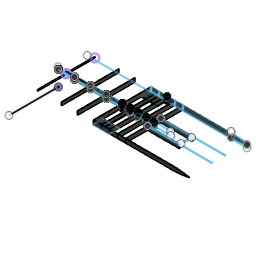
fishtail more cadamaran frame v4 (Autodesk Fusion 360 design; units mm, degrees)
Autodesk Fusion 360 part; units mm, degrees
sketch "Sketch1" plane through (0, 0, 0) normal (0, 1, 0) x (1, 0, 0)
  line L0 (0, 0, 0) -> (0, 0, -1544.9876)
  line L1 (2000, -550) -> (3000, -550)
  spline S0 degree 5 poles (0, -470) (19.8891, -472.7686) (59.6834, -478.151) (119.4225, -485.7607) (199.1707, -494.9751) (299.0134, -504.9326) (399.0022, -513.3461) (499.1108, -520.2801) (599.2925, -525.8722) (699.4727, -530.3612) (799.5726, -534.0348) (899.532, -537.1783) (999.3326, -540.0242) (1099.0214, -542.7014) (1198.7368, -545.1827) (1298.6488, -547.3474) (1398.9006, -549.0438) (1499.5491, -550.1503) (1600.504, -550.6385) (1701.4653, -550.6375) (1802.0225, -550.3661) (1881.8073, -550.1262) (1941.1238, -550.023) (1980.4165, -550) (2000, -550) knots 0 0 0 0 0 0 0.05 0.1 0.15 0.2 0.25 0.3 0.35 0.4 0.45 0.5 0.55 0.6 0.65 0.7 0.75 0.8 0.85 0.9 0.95 1 1 1 1 1 1
  line L2 (1800, -550) -> (2200, -550)
  spline S1 degree 5 poles (2000, -430) (1980.0012, -430) (1940.0021, -429.973) (1879.9994, -429.8512) (1799.9885, -429.5694) (1699.9671, -429.2542) (1599.9436, -429.2586) (1499.9235, -429.829) (1399.91, -431.0929) (1299.9035, -432.9733) (1199.9019, -435.2653) (1099.902, -437.7087) (999.901, -440.0615) (899.8967, -442.1718) (799.8896, -444.0523) (699.8815, -445.8304) (599.8751, -447.701) (499.8734, -449.8794) (399.8791, -452.5548) (299.8937, -455.8432) (199.9182, -459.8058) (119.9458, -463.5341) (59.9712, -466.6451) (19.99, -468.8585) (0, -470) knots 0 0 0 0 0 0 0.05 0.1 0.15 0.2 0.25 0.3 0.35 0.4 0.45 0.5 0.55 0.6 0.65 0.7 0.75 0.8 0.85 0.9 0.95 1 1 1 1 1 1
  line L3 (2204.0501, -430) -> (1795.9499, -430)
  line L4 (2000, -430) -> (3000, -430)
  line L5 (3000, -550) -> (3000, -430)
  point P0 (1500, -430)
  point P1 (500, -450)
  point P2 (500, -520)
  point P3 (1000, -540)
  point P4 (1500, -550)
  point P5 (1000, -440)
  constraint midpoint L1.start L2
  constraint midpoint S1.start L3
  constraint perpendicular L4 L5
  constraint coincident S0.start S1.end
extrude "Extrude1" add sketch "Sketch1" along normal mid plane 20 makes body 1
sketch "Sketch2" plane through (0, -10, 0) normal (0, -1, 0) x (1, 0, 0)
  spline S0 degree 5 poles (0, 470) (19.99, 468.8585) (59.9712, 466.6451) (119.9458, 463.5341) (199.9182, 459.8058) (299.8937, 455.8432) (399.8791, 452.5548) (499.8734, 449.8794) (599.8751, 447.701) (699.8815, 445.8304) (799.8896, 444.0523) (899.8967, 442.1718) (999.901, 440.0615) (1099.902, 437.7087) (1199.9019, 435.2653) (1299.9035, 432.9733) (1399.91, 431.0929) (1499.9235, 429.829) (1599.9436, 429.2586) (1699.9671, 429.2542) (1799.9885, 429.5694) (1879.9994, 429.8512) (1940.0021, 429.973) (1980.0012, 430) (2000, 430) knots -1 -1 -1 -1 -1 -1 -0.95 -0.9 -0.85 -0.8 -0.75 -0.7 -0.65 -0.6 -0.55 -0.5 -0.45 -0.4 -0.35 -0.3 -0.25 -0.2 -0.15 -0.1 -0.05 0 0 0 0 0 0
  line L0 (2000, 430) -> (3000, 430)
  line L1 (3000, 430) -> (3000, 550)
  line L2 (3000, 550) -> (2000, 550)
  spline S1 degree 5 poles (2000, 550) (1980.4165, 550) (1941.1238, 550.023) (1881.8073, 550.1262) (1802.0225, 550.3661) (1701.4653, 550.6375) (1600.504, 550.6385) (1499.5491, 550.1503) (1398.9006, 549.0438) (1298.6488, 547.3474) (1198.7368, 545.1827) (1099.0214, 542.7014) (999.3326, 540.0242) (899.532, 537.1783) (799.5726, 534.0348) (699.4727, 530.3612) (599.2925, 525.8722) (499.1108, 520.2801) (399.0022, 513.3461) (299.0134, 504.9326) (199.1707, 494.9751) (119.4225, 485.7607) (59.6834, 478.151) (19.8891, 472.7686) (0, 470) knots -1 -1 -1 -1 -1 -1 -0.95 -0.9 -0.85 -0.8 -0.75 -0.7 -0.65 -0.6 -0.55 -0.5 -0.45 -0.4 -0.35 -0.3 -0.25 -0.2 -0.15 -0.1 -0.05 0 0 0 0 0 0
  line L3 (3000, 550) -> (2990, 550)
  line L4 (2990, 550) -> (2990, 490)
  line L5 (2990, 490) -> (3000, 490)
  line L6 (3000, 490) -> (3000, 550)
  line L7 (3000, 550) -> (2750, 550)
  line L8 (2750, 550) -> (2500, 550)
  line L9 (2500, 550) -> (2250, 550)
  line L10 (2250, 550) -> (2000, 550)
  line L11 (2000, 550) -> (1750, 550)
  line L12 (1750, 550) -> (1500, 550)
  line L13 (1500, 550) -> (1250, 550)
  line L14 (1250, 550) -> (1000, 550)
  line L15 (1000, 550) -> (750, 550)
  line L16 (750, 550) -> (500, 550)
  line L17 (500, 550) -> (250, 550)
  line L18 (250, 550) -> (0, 550)
  line L19 (2750, 550) -> (2740, 550)
  line L20 (2740, 550) -> (2740, 490)
  line L21 (2740, 490) -> (2750, 490)
  line L22 (2750, 490) -> (2750, 550)
  line L23 (2500, 550) -> (2490, 550)
  line L24 (2490, 550) -> (2490, 490)
  line L25 (2490, 490) -> (2500, 490)
  line L26 (2500, 490) -> (2500, 550)
  line L27 (2250, 550) -> (2240, 550)
  line L28 (2240, 550) -> (2240, 500)
  line L29 (2240, 500) -> (2250, 500)
  line L30 (2250, 500) -> (2250, 550)
  line L31 (2000, 550) -> (1990, 550)
  line L32 (1990, 550) -> (1990, 490)
  line L33 (1990, 490) -> (2000, 490)
  line L34 (2000, 490) -> (2000, 550)
  line L35 (1500, 550) -> (1490, 550)
  line L36 (1490, 550) -> (1490, 490)
  line L37 (1490, 490) -> (1500, 490)
  line L38 (1500, 490) -> (1500, 550)
  line L39 (1000, 550) -> (990, 550)
  line L40 (990, 550) -> (990, 490)
  line L41 (990, 490) -> (1000, 490)
  line L42 (1000, 490) -> (1000, 550)
  line L43 (250, 510) -> (240, 510)
  line L44 (240, 510) -> (240, 480)
  line L45 (240, 480) -> (250, 480)
  line L46 (250, 480) -> (250, 510)
  line L47 (3000, 550) -> (2990, 550)
  line L48 (2990, 550) -> (2990, 430)
  line L49 (2990, 430) -> (3000, 430)
  line L50 (3000, 430) -> (3000, 550)
  line L51 (2750, 550) -> (2740, 550)
  line L52 (2740, 550) -> (2740, 430)
  line L53 (2740, 430) -> (2750, 430)
  line L54 (2750, 430) -> (2750, 550)
  line L55 (2500, 550) -> (2490, 550)
  line L56 (2490, 550) -> (2490, 430)
  line L57 (2490, 430) -> (2500, 430)
  line L58 (2500, 430) -> (2500, 550)
  line L59 (2250, 550) -> (2240, 550)
  line L60 (2240, 550) -> (2240, 430)
  line L61 (2240, 430) -> (2250, 430)
  line L62 (2250, 430) -> (2250, 550)
  line L63 (2000, 550) -> (2000, 430)
  line L64 (2000, 430) -> (1990, 430)
  line L65 (1990, 430) -> (1990, 550)
  line L66 (1990, 550) -> (2000, 550)
  line L67 (1500, 550) -> (1500, 430)
  line L68 (1500, 430) -> (1490, 430)
  line L69 (1490, 430) -> (1490, 550)
  line L70 (1490, 550) -> (1500, 550)
  line L71 (1000, 550) -> (1000, 430)
  line L72 (1000, 430) -> (990, 430)
  line L73 (990, 430) -> (990, 550)
  line L74 (990, 550) -> (1000, 550)
  line L75 (250, 520) -> (250, 450)
  line L76 (250, 450) -> (240, 450)
  line L77 (240, 450) -> (240, 520)
  line L78 (240, 520) -> (250, 520)
  line L79 (2245, 430) -> (2235.475, 430)
  line L80 (2245, 430) -> (2254.525, 430)
  line L81 (2254.525, 430) -> (2254.525, 449.05)
  line L82 (2235.475, 430) -> (2254.525, 430)
  line L83 (2254.525, 430) -> (2254.525, 449.05)
  line L84 (2254.525, 449.05) -> (2235.475, 449.05)
  line L85 (2235.475, 449.05) -> (2235.475, 430)
  constraint perpendicular L3 L4
  constraint parallel L3 L5
  constraint parallel L4 L6
  constraint coincident L2 L3.end
  constraint perpendicular L1 L3
  constraint coincident L1.end L2.start
  constraint perpendicular L4 L7
  constraint midpoint L2 L8.end
  constraint coincident L2 L9.end
  constraint parallel L2 L9
  constraint coincident L2.end S1.start
  constraint parallel L2 L10
  constraint parallel L2 L11
  constraint parallel L11 L12
  constraint parallel L12 L13
  constraint parallel L13 L14
  constraint parallel L14 L15
  constraint parallel L15 L16
  constraint parallel L16 L17
  constraint parallel L17 L18
  constraint horizontal L19
  constraint vertical L20
  constraint horizontal L21
  constraint vertical L22
  constraint horizontal L23
  constraint vertical L24
  constraint horizontal L25
  constraint vertical L26
  constraint horizontal L27
  constraint vertical L28
  constraint horizontal L29
  constraint vertical L30
  constraint horizontal L31
  constraint vertical L32
  constraint horizontal L33
  constraint vertical L34
  constraint horizontal L35
  constraint vertical L36
  constraint horizontal L37
  constraint vertical L38
  constraint horizontal L39
  constraint vertical L40
  constraint horizontal L41
  constraint vertical L42
  constraint horizontal L43
  constraint vertical L44
  constraint horizontal L45
  constraint vertical L46
  constraint horizontal L47
  constraint vertical L48
  constraint horizontal L49
  constraint vertical L50
  constraint coincident L0 L48.end
  constraint horizontal L51
  constraint vertical L52
  constraint horizontal L53
  constraint vertical L54
  constraint coincident L0 L52.end
  constraint horizontal L55
  constraint vertical L56
  constraint horizontal L57
  constraint vertical L58
  constraint coincident L0 L56.end
  constraint horizontal L59
  constraint vertical L60
  constraint horizontal L61
  constraint vertical L62
  constraint coincident L0 L60.end
  constraint perpendicular L63 L64
  constraint parallel L63 L65
  constraint parallel L64 L66
  constraint coincident S0.end L0.start
  constraint perpendicular L67 L68
  constraint parallel L67 L69
  constraint parallel L68 L70
  constraint coincident S0 L67.end
  constraint perpendicular L12 L67
  constraint perpendicular L71 L72
  constraint parallel L71 L73
  constraint parallel L72 L74
  constraint perpendicular L14 L71
  constraint perpendicular L75 L76
  constraint parallel L75 L77
  constraint parallel L76 L78
  constraint perpendicular L17 L75
  constraint midpoint L61 L79.start
  constraint parallel L0 L79
  constraint parallel L0 L80
  constraint perpendicular L80 L81
  constraint horizontal L82
  constraint vertical L83
  constraint horizontal L84
  constraint vertical L85
extrude "Extrude2" cut sketch "Sketch2" against normal blind 20 contours S1 L36 L37 L38 L67 L69 | L11 L31 L32 L33 L34 L63 L65 L66 | S1 L40 L41 L42 L71 L73 | L2 L10 L27 L28 L29 L30 L59 L60 L62 | S1 L44 L45 L46 L75 L77 | L2 L9 L23 L24 L25 L26 L55 L56 L58 | S1 L43 L44 L46 L75 L77 | L2 L8 L19 L20 L21 L22 L51 L52 L54 | L1 L2 L3 L4 L5 L6 L7 L47 L48 L50 bodies 1
extrude "Extrude3" add sketch "Sketch2" along normal blind 890 separate body contours S0 L33 L63 L64 L65 | S1 L11 L31 L32 L33 L34 L63 L65 L66 | L0 L60 L61 L62 L79 L80 L82 L84 | L29 L60 L62 L84 | L2 L10 L27 L28 L29 L30 L59 L60 L62 | L2 L9 L23 L24 L25 L26 L55 L56 L58 | L0 L25 L56 L57 L58 | L2 L8 L19 L20 L21 L22 L51 L52 L54 | L0 L21 L52 L53 L54 | L1 L2 L3 L4 L5 L6 L7 L47 L48 L50 | L0 L1 L5 L48 L49 L50 makes body 2 at (2490, -306.6667, 470) makes body 3 at (2740, -306.6667, 470) makes body 4 at (2990, -306.6667, 470) makes body 5 at (2250, -603.3333, 483.0167) makes body 6 at (1990, -306.6667, 450)
extrude "Extrude4" add sketch "Sketch2" against normal blind 20 contours S1 L11 L31 L32 L33 L34 L63 L65 L66 | L2 L10 L27 L28 L29 L30 L59 L60 L62 | L2 L9 L23 L24 L25 L26 L55 L56 L58 | L2 L8 L19 L20 L21 L22 L51 L52 L54 | L1 L2 L3 L4 L5 L6 L7 L47 L48 L50 bodies 4 3 5 2 6
sketch "Sketch3" plane through (0, 10, 0) normal (0, 1, 0) x (-1, 0, 0)
  line L0 (-2740, 550) -> (-2740, 490)
  line L1 (-2740, 490) -> (-2750, 490)
  line L2 (-2750, 490) -> (-2750, 550)
  line L3 (-2750, 550) -> (-2990, 550)
  line L4 (-2990, 550) -> (-2990, 490)
  line L5 (-2990, 490) -> (-3000, 490)
  line L6 (-3000, 490) -> (-3000, 430)
  line L7 (-3000, 430) -> (-2000, 430)
  spline S0 degree 5 poles (-2000, 430) (-1980.0012, 430) (-1940.0021, 429.973) (-1879.9994, 429.8512) (-1799.9885, 429.5694) (-1699.9671, 429.2542) (-1599.9436, 429.2586) (-1499.9235, 429.829) (-1399.91, 431.0929) (-1299.9035, 432.9733) (-1199.9019, 435.2653) (-1099.902, 437.7087) (-999.901, 440.0615) (-899.8967, 442.1718) (-799.8896, 444.0523) (-699.8815, 445.8304) (-599.8751, 447.701) (-499.8734, 449.8794) (-399.8791, 452.5548) (-299.8937, 455.8432) (-199.9182, 459.8058) (-119.9458, 463.5341) (-59.9712, 466.6451) (-19.99, 468.8585) (0, 470) knots 0 0 0 0 0 0 0.05 0.1 0.15 0.2 0.25 0.3 0.35 0.4 0.45 0.5 0.55 0.6 0.65 0.7 0.75 0.8 0.85 0.9 0.95 1 1 1 1 1 1
  spline S1 degree 5 poles (0, 470) (-19.8891, 472.7686) (-59.6834, 478.151) (-107.6487, 484.2609) (-155.6604, 489.9203) (-203.7179, 495.1274) (-231.8394, 498.0184) (-240, 498.8443) knots 0 0 0 0 0 0 0.05 0.1 0.120437 0.120437 0.120437 0.120437 0.120437 0.120437
  line L8 (-240, 498.8443) -> (-240, 480)
  line L9 (-240, 480) -> (-250, 480)
  line L10 (-250, 480) -> (-250, 499.8485)
  spline S2 degree 5 poles (-250, 499.8485) (-259.8064, 500.8255) (-289.5866, 503.7351) (-339.3666, 508.3088) (-409.1913, 514.0518) (-499.1108, 520.2801) (-599.2925, 525.8722) (-699.4727, 530.3612) (-797.7051, 533.9662) (-875.8104, 536.4321) (-933.8562, 538.138) (-971.9088, 539.217) (-990, 539.7219) knots 0.125445 0.125445 0.125445 0.125445 0.125445 0.125445 0.15 0.2 0.25 0.3 0.35 0.4 0.45 0.495336 0.495336 0.495336 0.495336 0.495336 0.495336
  line L11 (-990, 539.7219) -> (-990, 490)
  line L12 (-990, 490) -> (-1000, 490)
  line L13 (-1000, 490) -> (-1000, 540)
  spline S3 degree 5 poles (-1000, 540) (-1019.8114, 540.549) (-1059.5637, 541.6317) (-1119.2422, 543.2046) (-1198.8759, 545.1857) (-1296.7405, 547.3061) (-1375.0207, 548.6395) (-1433.4188, 549.3842) (-1471.7728, 549.7625) (-1490, 549.9178) knots 0.500348 0.500348 0.500348 0.500348 0.500348 0.500348 0.55 0.6 0.65 0.7 0.745225 0.745225 0.745225 0.745225 0.745225 0.745225
  line L14 (-1490, 549.9178) -> (-1490, 490)
  line L15 (-1490, 490) -> (-1500, 490)
  line L16 (-1500, 490) -> (-1500, 550)
  spline S4 degree 5 poles (-1500, 550) (-1520.0821, 550.1593) (-1560.3484, 550.4195) (-1620.847, 550.6383) (-1701.5404, 550.6373) (-1802.0225, 550.3661) (-1881.8073, 550.1262) (-1941.1238, 550.023) (-1980.4165, 550) (-2000, 550) knots 0.750187 0.750187 0.750187 0.750187 0.750187 0.750187 0.8 0.85 0.9 0.95 1 1 1 1 1 1
  line L17 (-2000, 550) -> (-1990, 550)
  line L18 (-1990, 550) -> (-1990, 490)
  line L19 (-1990, 490) -> (-2000, 490)
  line L20 (-2000, 490) -> (-2000, 550)
  line L21 (-2000, 550) -> (-2240, 550)
  line L22 (-2240, 550) -> (-2240, 500)
  line L23 (-2240, 500) -> (-2250, 500)
  line L24 (-2250, 500) -> (-2250, 550)
  line L25 (-2250, 550) -> (-2490, 550)
  line L26 (-2490, 550) -> (-2490, 490)
  line L27 (-2490, 490) -> (-2500, 490)
  line L28 (-2500, 490) -> (-2500, 550)
  line L29 (-2500, 550) -> (-2740, 550)
  line L30 (-3000, 550) -> (-2990, 550)
  line L31 (-2990, 550) -> (-2990, 430)
  line L32 (-2990, 430) -> (-3000, 430)
  line L33 (-3000, 430) -> (-3000, 550)
  line L34 (-2750, 550) -> (-2740, 550)
  line L35 (-2740, 550) -> (-2740, 430)
  line L36 (-2740, 430) -> (-2750, 430)
  line L37 (-2750, 430) -> (-2750, 550)
  line L38 (-2500, 550) -> (-2490, 550)
  line L39 (-2490, 550) -> (-2490, 430)
  line L40 (-2490, 430) -> (-2500, 430)
  line L41 (-2500, 430) -> (-2500, 550)
  line L42 (-2250, 550) -> (-2240, 550)
  line L43 (-2240, 550) -> (-2240, 430)
  line L44 (-2240, 430) -> (-2250, 430)
  line L45 (-2250, 430) -> (-2250, 550)
  line L46 (-2000, 550) -> (-1990, 550)
  line L47 (-1990, 550) -> (-1990, 429.9986)
  line L48 (-1990, 429.9986) -> (-2000, 429.9986)
  line L49 (-2000, 429.9986) -> (-2000, 550)
  line L50 (-1500, 550) -> (-1490, 550)
  line L51 (-1490, 550) -> (-1490, 430)
  line L52 (-1490, 430) -> (-1500, 430)
  line L53 (-1500, 430) -> (-1500, 550)
  line L54 (-1000, 550) -> (-990, 550)
  line L55 (-990, 550) -> (-990, 430)
  line L56 (-990, 430) -> (-1000, 430)
  line L57 (-1000, 430) -> (-1000, 550)
  line L58 (-250, 510) -> (-240, 510)
  line L59 (-240, 510) -> (-240, 450)
  line L60 (-240, 450) -> (-250, 450)
  line L61 (-250, 450) -> (-250, 510)
  spline S5 degree 5 poles (0, 470) (-19.8891, 472.7686) (-59.6834, 478.151) (-119.4225, 485.7607) (-199.1707, 494.9751) (-299.0134, 504.9326) (-399.0022, 513.3461) (-499.1108, 520.2801) (-599.2925, 525.8722) (-699.4727, 530.3612) (-799.5726, 534.0348) (-899.532, 537.1783) (-999.3326, 540.0242) (-1099.0214, 542.7014) (-1198.7368, 545.1827) (-1298.6488, 547.3474) (-1398.9006, 549.0438) (-1499.5491, 550.1503) (-1600.504, 550.6385) (-1701.4653, 550.6375) (-1802.0225, 550.3661) (-1881.8073, 550.1262) (-1941.1238, 550.023) (-1980.4165, 550) (-2000, 550) knots 0 0 0 0 0 0 0.05 0.1 0.15 0.2 0.25 0.3 0.35 0.4 0.45 0.5 0.55 0.6 0.65 0.7 0.75 0.8 0.85 0.9 0.95 1 1 1 1 1 1
  line L62 (-1800, 550) -> (-2200, 550)
  spline S6 degree 5 poles (-2000, 430) (-1980.0012, 430) (-1940.0023, 429.973) (-1879.9999, 429.8518) (-1799.9893, 429.5709) (-1699.9683, 429.2567) (-1599.9453, 429.2609) (-1499.9254, 429.8294) (-1399.9123, 431.0898) (-1299.9061, 432.9666) (-1199.9048, 435.2567) (-1099.9054, 437.7018) (-999.9049, 440.0605) (-899.9012, 442.1804) (-799.8947, 444.071) (-699.8871, 445.8553) (-599.8811, 447.7229) (-499.8794, 449.8839) (-399.8848, 452.5233) (-299.8987, 455.7547) (-199.922, 459.638) (-119.9483, 463.2847) (-59.9725, 466.3244) (-19.9905, 468.4856) (0, 469.6) knots 0 0 0 0 0 0 0.05 0.1 0.15 0.2 0.25 0.3 0.35 0.4 0.45 0.5 0.55 0.6 0.65 0.7 0.75 0.8 0.85 0.9 0.95 1 1 1 1 1 1
  line L63 (-2204.0501, 430) -> (-1795.9499, 430)
  spline S7 degree 5 poles (0, 470) (-19.8891, 472.7686) (-59.6834, 478.151) (-119.4225, 485.7607) (-199.1707, 494.9751) (-299.0134, 504.9326) (-399.0022, 513.3461) (-499.1108, 520.2801) (-599.2925, 525.8722) (-699.4727, 530.3612) (-799.5726, 534.0348) (-899.532, 537.1783) (-999.3326, 540.0242) (-1099.0214, 542.7014) (-1198.7368, 545.1827) (-1298.6488, 547.3474) (-1398.9006, 549.0438) (-1499.5491, 550.1503) (-1600.504, 550.6385) (-1701.4653, 550.6375) (-1802.0225, 550.3661) (-1881.8073, 550.1262) (-1941.1238, 550.023) (-1980.4165, 550) (-2000, 550) knots 0 0 0 0 0 0 0.05 0.1 0.15 0.2 0.25 0.3 0.35 0.4 0.45 0.5 0.55 0.6 0.65 0.7 0.75 0.8 0.85 0.9 0.95 1 1 1 1 1 1
  line L64 (-1800, 550) -> (-2200, 550)
  spline S8 degree 5 poles (-2000, 430) (-1980.0012, 430) (-1940.0023, 429.973) (-1879.9999, 429.8518) (-1799.9893, 429.5709) (-1699.9683, 429.2567) (-1599.9453, 429.2609) (-1499.9254, 429.8294) (-1399.9123, 431.0898) (-1299.9061, 432.9666) (-1199.9048, 435.2567) (-1099.9054, 437.7018) (-999.9049, 440.0605) (-899.9012, 442.1804) (-799.8947, 444.071) (-699.8871, 445.8553) (-599.8811, 447.7229) (-499.8794, 449.8839) (-399.8848, 452.5233) (-299.8987, 455.7547) (-199.922, 459.638) (-119.9483, 463.2847) (-59.9725, 466.3244) (-19.9905, 468.4856) (0, 469.6) knots 0 0 0 0 0 0 0.05 0.1 0.15 0.2 0.25 0.3 0.35 0.4 0.45 0.5 0.55 0.6 0.65 0.7 0.75 0.8 0.85 0.9 0.95 1 1 1 1 1 1
  line L65 (-2204.0501, 430) -> (-1795.9499, 430)
  spline S9 degree 5 poles (0, 470) (-19.8891, 472.7686) (-59.6834, 478.151) (-119.4225, 485.7607) (-199.1707, 494.9751) (-299.0134, 504.9326) (-399.0022, 513.3461) (-499.1108, 520.2801) (-599.2925, 525.8722) (-699.4727, 530.3612) (-799.5726, 534.0348) (-899.532, 537.1783) (-999.3326, 540.0242) (-1099.0214, 542.7014) (-1198.7368, 545.1827) (-1298.6488, 547.3474) (-1398.9006, 549.0438) (-1499.5491, 550.1503) (-1600.504, 550.6385) (-1701.4653, 550.6375) (-1802.0225, 550.3661) (-1881.8073, 550.1262) (-1941.1238, 550.023) (-1980.4165, 550) (-2000, 550) knots 0 0 0 0 0 0 0.05 0.1 0.15 0.2 0.25 0.3 0.35 0.4 0.45 0.5 0.55 0.6 0.65 0.7 0.75 0.8 0.85 0.9 0.95 1 1 1 1 1 1
  line L66 (-1800, 550) -> (-2200, 550)
  spline S10 degree 5 poles (-2000, 430) (-1980.0012, 430) (-1940.0023, 429.973) (-1879.9999, 429.8518) (-1799.9893, 429.5709) (-1699.9683, 429.2567) (-1599.9453, 429.2609) (-1499.9254, 429.8294) (-1399.9123, 431.0898) (-1299.9061, 432.9666) (-1199.9048, 435.2567) (-1099.9054, 437.7018) (-999.9049, 440.0605) (-899.9012, 442.1804) (-799.8947, 444.071) (-699.8871, 445.8553) (-599.8811, 447.7229) (-499.8794, 449.8839) (-399.8848, 452.5233) (-299.8987, 455.7547) (-199.922, 459.638) (-119.9483, 463.2847) (-59.9725, 466.3244) (-19.9905, 468.4856) (0, 469.6) knots 0 0 0 0 0 0 0.05 0.1 0.15 0.2 0.25 0.3 0.35 0.4 0.45 0.5 0.55 0.6 0.65 0.7 0.75 0.8 0.85 0.9 0.95 1 1 1 1 1 1
  line L67 (-2204.0501, 430) -> (-1795.9499, 430)
  line L68 (-2000, 550) -> (-3500, 550)
  line L69 (-2000, 430) -> (-3500, 430)
  spline S11 degree 5 poles (0, 470) (-19.8891, 472.7686) (-59.6834, 478.151) (-119.4225, 485.7607) (-199.1707, 494.9751) (-299.0134, 504.9326) (-399.0022, 513.3461) (-499.1108, 520.2801) (-599.2925, 525.8722) (-699.4727, 530.3612) (-799.5726, 534.0348) (-899.532, 537.1783) (-999.3326, 540.0242) (-1099.0214, 542.7014) (-1198.7368, 545.1827) (-1298.6488, 547.3474) (-1398.9006, 549.0438) (-1499.5491, 550.1503) (-1600.504, 550.6385) (-1701.4653, 550.6375) (-1802.0225, 550.3661) (-1881.8073, 550.1262) (-1941.1238, 550.023) (-1980.4165, 550) (-2000, 550) knots 0 0 0 0 0 0 0.05 0.1 0.15 0.2 0.25 0.3 0.35 0.4 0.45 0.5 0.55 0.6 0.65 0.7 0.75 0.8 0.85 0.9 0.95 1 1 1 1 1 1
  line L70 (-1800, 550) -> (-2200, 550)
  spline S12 degree 5 poles (-2000, 430) (-1980.0012, 430) (-1940.0023, 429.973) (-1879.9999, 429.8518) (-1799.9893, 429.5709) (-1699.9683, 429.2567) (-1599.9453, 429.2609) (-1499.9254, 429.8294) (-1399.9123, 431.0898) (-1299.9061, 432.9666) (-1199.9048, 435.2567) (-1099.9054, 437.7018) (-999.9049, 440.0605) (-899.9012, 442.1804) (-799.8947, 444.071) (-699.8871, 445.8553) (-599.8811, 447.7229) (-499.8794, 449.8839) (-399.8848, 452.5233) (-299.8987, 455.7547) (-199.922, 459.638) (-119.9483, 463.2847) (-59.9725, 466.3244) (-19.9905, 468.4856) (0, 469.6) knots 0 0 0 0 0 0 0.05 0.1 0.15 0.2 0.25 0.3 0.35 0.4 0.45 0.5 0.55 0.6 0.65 0.7 0.75 0.8 0.85 0.9 0.95 1 1 1 1 1 1
  line L71 (-2204.0501, 430) -> (-1795.9499, 430)
  line L72 (-2250, 500) -> (-2240, 500)
  line L73 (-2240, 410) -> (-2240, 500)
  line L74 (-2250, 500) -> (-2250, 410)
  line L75 (-2250, 430) -> (-2240, 430)
  line L76 (-2250, 500) -> (-2240, 500)
  line L77 (-2240, 500) -> (-2240, 430)
  line L78 (-2240, 430) -> (-2250, 430)
  line L79 (-2250, 430) -> (-2250, 500)
  line L80 (-2250, 500) -> (-2240, 500)
  line L81 (-2240, 500) -> (-2240, 430)
  line L82 (-2240, 430) -> (-2250, 430)
  line L83 (-2250, 430) -> (-2250, 500)
  line L84 (-2000, 490) -> (-1990, 490)
  line L85 (-1990, 490) -> (-1990, 429.9986)
  line L86 (-1990, 429.9986) -> (-2000, 429.9986)
  line L87 (-2000, 429.9986) -> (-2000, 490)
  point P0 (-1500, 430)
  point P1 (-500, 450)
  point P2 (-500, 520)
  point P3 (-1000, 540)
  point P4 (-1500, 550)
  point P5 (-1000, 440)
  point P6 (-1500, 430)
  point P7 (-500, 450)
  point P8 (-500, 520)
  point P9 (-1000, 540)
  point P10 (-1500, 550)
  point P11 (-1000, 440)
  point P12 (-1500, 430)
  point P13 (-500, 450)
  point P14 (-500, 520)
  point P15 (-1000, 540)
  point P16 (-1500, 550)
  point P17 (-1000, 440)
  point P18 (-1500, 430)
  point P19 (-500, 450)
  point P20 (-500, 520)
  point P21 (-1000, 540)
  point P22 (-1500, 550)
  point P23 (-1000, 440)
  constraint perpendicular L30 L31
  constraint parallel L30 L32
  constraint parallel L31 L33
  constraint coincident L3.end L4.start
  constraint perpendicular L4 L30
  constraint perpendicular L34 L35
  constraint parallel L34 L36
  constraint parallel L35 L37
  constraint coincident L0.start L29.end
  constraint perpendicular L0 L34
  constraint coincident L2.end L3.start
  constraint perpendicular L38 L39
  constraint parallel L38 L40
  constraint parallel L39 L41
  constraint coincident L25.end L26.start
  constraint perpendicular L26 L38
  constraint coincident L28.end L29.start
  constraint perpendicular L42 L43
  constraint parallel L42 L44
  constraint parallel L43 L45
  constraint coincident L21.end L22.start
  constraint perpendicular L22 L42
  constraint coincident L24.end L25.start
  constraint perpendicular L46 L47
  constraint parallel L46 L48
  constraint parallel L47 L49
  constraint coincident L17.end L18.start
  constraint coincident S4.end L17.start
  constraint perpendicular L50 L51
  constraint parallel L50 L52
  constraint parallel L51 L53
  constraint perpendicular L16 L50
  constraint coincident P16 P10
  constraint horizontal L54
  constraint vertical L55
  constraint horizontal L56
  constraint vertical L57
  constraint horizontal L58
  constraint vertical L59
  constraint horizontal L60
  constraint vertical L61
  constraint midpoint S4.end L62
  constraint midpoint L7.end L63
  constraint midpoint S4.end L64
  constraint midpoint L7.end L65
  constraint midpoint S4.end L66
  constraint midpoint L7.end L67
  constraint midpoint S4.end L70
  constraint midpoint L7.end L71
  constraint parallel L69 L71
  constraint coincident L23.end L24.start
  constraint coincident L22.end L23.start
  constraint perpendicular L72 L73
  constraint perpendicular L72 L74
  constraint horizontal L76
  constraint vertical L77
  constraint horizontal L78
  constraint vertical L79
  constraint horizontal L80
  constraint vertical L81
  constraint horizontal L82
  constraint vertical L83
  constraint horizontal L84
  constraint vertical L85
  constraint horizontal L86
  constraint vertical L87
  constraint coincident L19.end L20.start
extrude "Extrude5" add sketch "Sketch3" along normal blind 890 contours L0 L1 L2 L34 L35 L37 L68 | L1 L7 L35 L36 L37 L69 | L26 L27 L28 L38 L39 L41 L68 | L7 L27 L39 L40 L41 L69 | L4 L5 L30 L31 L33 L68 | L5 L6 L7 L31 L32 L33 L69 bodies 2 3 4
extrude "Extrude6" add 1 faces at (1993.3333, 10, 530.0004) along direction (0, 1, 0) blind 890 on bodies 6 bodies 6
extrude "Extrude7" add 1 faces at (2243.3333, 10, 516.6667) along direction (0, 1, 0) blind 890 on bodies 5 bodies 5
extrude "Extrude8" add 2 faces at (2243.3333, -10, 476.6667) (1993.3333, -10, 470) along direction (0, 1, 0) blind 20 and the other way blind -910 on bodies 5 6 bodies 5 6
extrude "Extrude9" add sketch "Sketch2" along normal blind 890 separate body contours S0 L37 L67 L69 | S1 L36 L37 L38 L67 L69 | S0 L41 L71 L73 | S1 L40 L41 L42 L71 L73 | S0 L45 L75 L77 | S1 L44 L45 L46 L75 L77 makes body 7 at (1500, -306.6667, 510) makes body 8 at (1000, -306.6667, 506.6667) makes body 9 at (250, -306.6667, 485.8678)
extrude "Extrude10" add sketch "Sketch2" against normal blind 910 contours S1 L36 L37 L38 L67 L69 | S1 L40 L41 L42 L71 L73 | S1 L44 L45 L46 L75 L77 bodies 7 8 9
extrude "Extrude11" add sketch "Sketch2" along normal blind -20 and the other way blind 910 contours S0 L37 L67 L69 | S0 L41 L71 L73 | S0 L45 L75 L77 bodies 7 8 9
sketch "Sketch4" plane through (240, 0, 0) normal (-1, 0, 0) x (0, -1, 0)
  line L0 (10, 480) -> (10, 458.3068)
  line L1 (10, 458.3068) -> (900, 458.3068)
  line L2 (900, 458.3068) -> (900, 498.8443)
  line L3 (900, 498.8443) -> (-900, 498.8443)
  line L4 (-900, 498.8443) -> (-900, 458.3068)
  line L5 (-900, 458.3068) -> (-10, 458.3068)
  line L6 (-10, 458.3068) -> (-10, 480)
  line L7 (-10, 480) -> (10, 480)
sketch "Sketch5" plane through (0, 0, 430) normal (0, 0, -1) x (1, 0, 0)
  line L0 (2500, -10) -> (2490, -10)
  line L1 (2490, -10) -> (2490, -900)
  line L2 (2490, -900) -> (2500, -900)
  line L3 (2500, -900) -> (2500, -10)
  line L4 (2500, -900) -> (2500, -600)
  line L5 (2500, -600) -> (1990, -600)
  line L6 (1990, -600) -> (1990, -900)
  line L7 (1990, -900) -> (2500, -900)
  line L8 (2500, 900) -> (2500, 600)
  line L9 (2500, 600) -> (1990, 600)
  line L10 (1990, 600) -> (1990, 900)
  line L11 (1990, 900) -> (2500, 900)
  constraint perpendicular L4 L5
  constraint parallel L4 L6
  constraint parallel L5 L7
  constraint perpendicular L2 L4
  constraint coincident L2.end L3.start
  constraint perpendicular L8 L9
  constraint parallel L8 L10
  constraint parallel L9 L11
  constraint vertical L8
extrude "Extrude12" cut sketch "Sketch5" against normal blind 10 contours L1 L2 L3 L4 L5 L7 | L1 L5 L6 L7 | L8 L9 L10 L11 bodies 5 2 6
extrude "Extrude13" add sketch "Sketch5" against normal blind 10 separate body contours L1 L2 L3 L4 L5 L7 | L1 L5 L6 L7 | L8 L9 L10 L11 makes body 10 at (2160, -800, 430) makes body 11 at (2160, 700, 430)
sketch "Sketch6" plane through (0, 900, 0) normal (0, 1, 0) x (-1, 0, 0)
  line L0 (-2500, 440) -> (-2490, 440)
  line L1 (-2490, 440) -> (-2490, 550)
  line L2 (-2490, 550) -> (-2500, 550)
  line L3 (-2500, 550) -> (-2500, 440)
  line L4 (0, 400) -> (-5000, 400)
  line L5 (-1990, 550) -> (-1990, 430)
  line L6 (-1990, 430) -> (-5000, 430)
  line L7 (-5000, 430) -> (-5000, 550)
  line L8 (-5000, 550) -> (-1990, 550)
  line L9 (-2500, 430) -> (-1990, 430)
  line L10 (-1990, 430) -> (-1990, 440)
  line L11 (-1990, 440) -> (-2500, 440)
  line L12 (-2500, 440) -> (-2500, 430)
  line L13 (-2240, 440) -> (-2250, 440)
  line L14 (-2000, 440) -> (-1990, 440)
  line L15 (-1990, 440) -> (-1990, 495)
  line L16 (-2750, 430) -> (-2740, 430)
  line L17 (-2740, 430) -> (-2740, 490)
  line L18 (-2740, 490) -> (-2750, 490)
  line L19 (-2750, 490) -> (-2750, 430)
  line L20 (-3000, 430) -> (-2990, 430)
  line L21 (-2990, 430) -> (-2990, 490)
  line L22 (-2990, 490) -> (-3000, 490)
  line L23 (-3000, 490) -> (-3000, 430)
  line L24 (-2500, 550) -> (-2490, 550)
  line L25 (-2490, 550) -> (-2490, 500)
  line L26 (-2490, 500) -> (-2500, 500)
  line L27 (-2500, 500) -> (-2500, 550)
  line L28 (-2250, 550) -> (-2240, 550)
  line L29 (-2240, 550) -> (-2240, 500)
  line L30 (-2240, 500) -> (-2250, 500)
  line L31 (-2250, 500) -> (-2250, 550)
  line L32 (-2000, 550) -> (-1990, 550)
  line L33 (-1990, 550) -> (-1990, 500)
  line L34 (-1990, 500) -> (-2000, 500)
  line L35 (-2000, 500) -> (-2000, 550)
  line L36 (-3000, 490) -> (-2990, 490)
  line L37 (-2990, 490) -> (-2990, 550)
  line L38 (-2990, 550) -> (-3000, 550)
  line L39 (-3000, 550) -> (-3000, 490)
  line L40 (-2750, 490) -> (-2740, 490)
  line L41 (-2740, 490) -> (-2740, 550)
  line L42 (-2740, 550) -> (-2750, 550)
  line L43 (-2750, 550) -> (-2750, 490)
  line L44 (-2500, 500) -> (-2490, 500)
  line L45 (-2490, 500) -> (-2490, 440)
  line L46 (-2490, 440) -> (-2500, 440)
  line L47 (-2500, 440) -> (-2500, 500)
  line L48 (-2250, 500) -> (-2240, 500)
  line L49 (-2240, 500) -> (-2240, 440)
  line L50 (-2240, 440) -> (-2250, 440)
  line L51 (-2250, 440) -> (-2250, 500)
  line L52 (-2000, 500) -> (-1990, 500)
  line L53 (-1990, 500) -> (-1990, 440)
  line L54 (-1990, 440) -> (-2000, 440)
  line L55 (-2000, 440) -> (-2000, 500)
  spline S0 degree 5 poles (-4500, 550) (-4517.603, 550) (-4554.0378, 549.2689) (-4612.3723, 545.9812) (-4696.0644, 537.8448) (-4804.1552, 523.6896) (-4887.7976, 510.6722) (-4946.0615, 500.4661) (-4982.4328, 493.5134) (-5000, 490) knots 0 0 0 0 0 0 0.2 0.4 0.6 0.8 1 1 1 1 1 1
  line L56 (-4450, 550) -> (-4550, 550)
  spline S1 degree 5 poles (-4500, 430) (-4519.7205, 430) (-4559.3098, 430.6716) (-4619.1383, 433.6921) (-4699.6212, 441.214) (-4800.6249, 454.6612) (-4881.0519, 467.6513) (-4940.8014, 478.4224) (-4980.3196, 486.0639) (-5000, 490) knots 0 0 0 0 0 0 0.2 0.4 0.6 0.8 1 1 1 1 1 1
  line L57 (-4450, 430) -> (-4550, 430)
  line L58 (-4500, 550) -> (-4500, 600)
  line L59 (-4950, 480) -> (-5050, 500)
  line L60 (-4950, 500) -> (-5050, 480)
  constraint horizontal L4
  constraint perpendicular L5 L6
  constraint parallel L5 L7
  constraint parallel L6 L8
  constraint vertical L5
  constraint horizontal L9
  constraint vertical L10
  constraint horizontal L11
  constraint vertical L12
  constraint coincident L5 L10.end
  constraint coincident L6 L9.start
  constraint coincident L11 L13.end
  constraint horizontal L14
  constraint vertical L15
  constraint coincident L5 L15.end
  constraint coincident L11 L14.start
  constraint horizontal L16
  constraint vertical L17
  constraint horizontal L18
  constraint vertical L19
  constraint coincident L6 L16.start
  constraint horizontal L20
  constraint vertical L21
  constraint horizontal L22
  constraint vertical L23
  constraint coincident L6 L20.start
  constraint horizontal L24
  constraint vertical L25
  constraint horizontal L26
  constraint vertical L27
  constraint coincident L1 L25.end
  constraint coincident L2.end L3.start
  constraint horizontal L28
  constraint vertical L29
  constraint horizontal L30
  constraint vertical L31
  constraint coincident L8 L28.start
  constraint horizontal L32
  constraint vertical L33
  constraint horizontal L34
  constraint vertical L35
  constraint coincident L5 L33.end
  constraint coincident L8 L32.start
  constraint horizontal L36
  constraint vertical L37
  constraint horizontal L38
  constraint vertical L39
  constraint coincident L8 L37.end
  constraint horizontal L40
  constraint vertical L41
  constraint horizontal L42
  constraint vertical L43
  constraint coincident L8 L41.end
  constraint horizontal L44
  constraint vertical L45
  constraint horizontal L46
  constraint vertical L47
  constraint coincident L0.end L1.start
  constraint horizontal L48
  constraint vertical L49
  constraint horizontal L50
  constraint vertical L51
  constraint horizontal L52
  constraint vertical L53
  constraint horizontal L54
  constraint vertical L55
  constraint midpoint S0.start L56
  constraint midpoint S1.start L57
  constraint coincident L8 S0.start
  constraint perpendicular L8 L58
  constraint coincident L6 S1.start
  constraint midpoint S0.end L59
  constraint midpoint S0.end L60
extrude "Extrude14" cut sketch "Sketch6" against normal blind 10 contours L0 L1 L3 L11 L26 L44 L45 L46 L47 | L11 L13 L30 L48 L49 L50 L51 | L8 L18 L40 L41 L42 L43 | L5 L11 L14 L15 L34 L52 L53 L54 L55 | L8 L22 L36 L37 L38 L39 bodies 4 3 5 2 6
extrude "Extrude15" add sketch "Sketch6" against normal blind 10 separate body contours L0 L1 L3 L11 L26 L44 L45 L46 L47 | L3 L6 L8 L12 L17 L27 L41 L47 | L1 L8 L11 L25 L31 L45 L51 | L11 L13 L30 L48 L49 L50 L51 | L8 L11 L29 L35 L49 L55 | L8 L18 L40 L41 L42 L43 | L5 L11 L14 L15 L34 L52 L53 L54 L55 | L6 L8 L19 L21 L37 L43 | L8 L22 L36 L37 L38 L39 | L6 L8 L23 L39 S0 L56 S1 L57 makes body 12
mirror "Mirror1" about plane through (0, 0, 0) normal (0, 1, 0) of bodies 12 makes body 13
extrude "Extrude16" cut sketch "Sketch2" along normal blind 880 and the other way blind 900 contours L0 L60 L79 L82 L84 L85 | L0 L60 L61 L62 L79 L80 L82 L84 | L0 L62 L80 L81 L82 L83 L84 bodies 5 10 11
extrude "Extrude17" add sketch "Sketch2" along normal blind 880 and the other way blind 900 separate body contours L0 L60 L79 L82 L84 L85 | L0 L60 L61 L62 L79 L80 L82 L84 | L0 L62 L80 L81 L82 L83 L84 makes body 14
extrude "Extrude18" cut sketch "Sketch2" against normal blind 20 contours L0 L60 L79 L82 L84 L85 | L0 L60 L61 L62 L79 L80 L82 L84 | L0 L62 L80 L81 L82 L83 L84 bodies 1
mirror "Mirror2" about plane through (0, 0, 0) normal (0, 1, 0) of "Extrude14"
sketch "Sketch7" plane through (0, 0, 550) normal (0, 0, 1) x (-1, 0, 0)
  line L0 (-2990, 890) -> (-3000, 890)
  line L1 (-3000, 890) -> (-3000, -890)
  line L2 (-3000, -890) -> (-2990, -890)
  line L3 (-2990, -890) -> (-2990, 890)
  line L4 (-4000, 0) -> (-4000, -163.83)
  line L5 (-4000, 0) -> (-4000, 163.83)
  line L6 (-4000, -200) -> (-4000, 200)
  line L7 (-4000, -200) -> (-4000, -210)
  line L8 (-4000, 200) -> (-4000, 210)
  line L9 (-4000, 200) -> (-2990, 200)
  line L10 (-2990, 210) -> (-4000, 210)
  line L11 (-4000, -210) -> (-2990, -210)
  line L12 (-2990, -200) -> (-4000, -200)
  line L13 (-4000, 200) -> (-5000, 200)
  line L14 (-5000, 200) -> (-5000, 210)
  line L15 (-5000, 210) -> (-4000, 210)
  line L16 (-4000, 210) -> (-4000, 200)
  line L17 (-4000, -210) -> (-5000, -210)
  line L18 (-5000, -210) -> (-5000, -200)
  line L19 (-5000, -200) -> (-4000, -200)
  line L20 (-4000, -200) -> (-4000, -210)
  line L21 (-3000, 200) -> (-3000, 210)
  line L22 (-3000, -210) -> (-3000, -200)
  line L23 (-4000, 210) -> (-2990, 210)
  constraint vertical L4
  constraint parallel L4 L5
  constraint parallel L4 L6
  constraint vertical L7
  constraint vertical L8
  constraint coincident L3 L9.end
  constraint perpendicular L3 L9
  constraint coincident L3 L10.start
  constraint perpendicular L8 L10
  constraint coincident L3 L11.end
  constraint perpendicular L3 L11
  constraint coincident L3 L12.start
  constraint perpendicular L6 L12
  constraint horizontal L13
  constraint vertical L14
  constraint horizontal L15
  constraint vertical L16
  constraint horizontal L17
  constraint vertical L18
  constraint horizontal L19
  constraint vertical L20
  constraint coincident L9 L21.start
  constraint coincident L1 L21.start
  constraint coincident L10 L21.end
  constraint coincident L1 L21.end
  constraint coincident L11 L22.start
  constraint coincident L1 L22.start
  constraint coincident L12 L22.end
  constraint coincident L1 L22.end
extrude "Extrude25" add sketch "Sketch7" against normal blind 120 separate body contours L1 L8 L9 L10 L16 L21 L23 | L1 L7 L11 L12 L20 L22 makes body 15 at (3666.6667, 210, 510) makes body 16 at (3666.6667, -200, 510)
extrude "Extrude26" cut sketch "Sketch7" against normal blind 60 contours L1 L3 L9 L10 L21 L23 | L1 L3 L11 L12 L22 bodies 4
extrude "Extrude19" [suppressed]
extrude "Extrude20" [suppressed]
extrude "Extrude21" [suppressed]
extrude "Extrude22" [suppressed]
extrude "Extrude23" [suppressed]
extrude "Extrude24" [suppressed]
